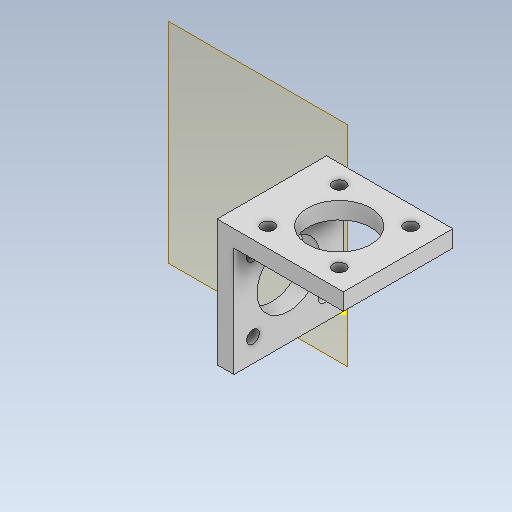
# Autodesk Inventor part: base_1
Saved by Autodesk Inventor 2020 (Build 240168000, 168)
## iProperties
Created: 2022-01-18
Part Number: base_1
Material: Generic
Document SubType Name: Modeling
Designer: Shuang Peng
Density: 1 g/cm^3
Appearance: Default
Author: Shuang Peng
Autodesk Inventor part; units mm, degrees
ref_plane "YZ Plane" through (0, 0, 0) normal (1, 0, 0) x (0, 1, 0)
ref_plane "XZ Plane" through (0, 0, 0) normal (0, 1, 0) x (-1, 0, 0)
ref_plane "XY Plane" through (0, 0, 0) normal (0, 0, 1) x (1, 0, 0)
ref_plane "Work Plane1" through (-18.4246, 0, 0) normal (0, 0, 1) x (1, 0, 0)
sketch "Sketch1" plane through (-18.4246, 0, 0) normal (0, 0, 1) x (1, 0, 0)
  line L0 (0, -0.9373) -> (0, 15) projected
  line L1 (0, 15) -> (15.9373, 15) projected
  line L2 (0, -0.9373) -> (0, 19.0627)
  line L3 (15.9373, 15) -> (-4.0627, 15)
  line L4 (0, 15) -> (2, 15)
  line L5 (2, 15) -> (2, 0)
  line L6 (2, 0) -> (0, 0)
  line L7 (0, 0) -> (0, 15)
  line L8 (0, 15) -> (15, 15)
  line L9 (15, 15) -> (15, 13)
  line L10 (15, 13) -> (0, 13)
  line L11 (0, 13) -> (0, 15)
  point P0 (18.4246, 0)
  point P1 (0, 0)
  point P2 (2, 13)
  point P3 (15, 15)
  dimension "d0" = 20
  dimension "d1" = 20
  dimension "d2" = 2
  dimension "d3" = 15
  dimension "d4" = 15
  dimension "d5" = 2
  constraints: 20 end point, 4 parallel, 2 horizontal, 2 perpendicular, 2 point on line
  measures "d0" distance of L0.start L2.end
  measures "d1" distance of L1.end L3.end
  measures "d2" distance of L5.end L6.end
  measures "d3" distance of L4.end L5.end
  measures "d4" distance of L9.end L10.end
  measures "d5" distance of L8.end L9.end
extrude "Extrusion1" add sketch "Sketch1" along normal blind 13
sketch "Sketch2" plane through (-16.4246, 0, 0) normal (1, 0, 0) x (0, 0, -1)
  circle A0 centre (-10.7426, 2.7574) radius 0.75 projected
  circle A1 centre (-10.7426, 11.2426) radius 0.75 projected
  circle A2 centre (-2.2574, 2.7574) radius 0.75 projected
  circle A3 centre (-2.2574, 11.2426) radius 0.75 projected
  point P0 (0, 0)
extrude "Extrusion2" cut sketch "Sketch2" against normal blind 13
sketch "Sketch3" plane through (-16.4246, 13, 0) normal (0, -1, 0) x (1, 0, 0)
  circle A0 centre (1.7574, 10.7426) radius 0.75 projected
  circle A1 centre (10.2426, 10.7426) radius 0.75 projected
  circle A2 centre (10.2426, 2.2574) radius 0.75 projected
  circle A3 centre (1.7574, 2.2574) radius 0.75 projected
  point P0 (16.4246, 0)
extrude "Extrusion3" cut sketch "Sketch3" against normal blind 13
sketch "Sketch4" plane through (-16.4246, 0, 0) normal (1, 0, 0) x (0, 0, -1)
  point P0 (0, 0)
sketch "Sketch5" plane through (-16.4246, 0, 0) normal (1, 0, 0) x (0, 0, -1)
  circle A0 centre (-6.5, 7) radius 1.5 projected
  circle A1 centre (-6.5, 7) radius 3.75
  point P0 (0, 0)
  dimension "d12" = 7.5
  constraints: 1 centre point, 1 coincident
  measures "d12" diameter of A1
extrude "Extrusion4" cut sketch "Sketch5" against normal blind 13 contours A0 | A1
sketch "Sketch6" plane through (-16.4246, 13, 0) normal (0, -1, 0) x (1, 0, 0)
  circle A0 centre (6, 6.5) radius 1.5 projected
  circle A1 centre (6, 6.5) radius 3.75
  point P0 (16.4246, 0)
  dimension "d15" = 7.5
  constraints: 1 centre point, 1 coincident
  measures "d15" diameter of A1
extrude "Extrusion5" cut sketch "Sketch6" against normal blind 13 contours A0 | A1
body "Solid1"
